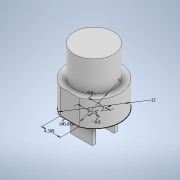
# Autodesk Inventor part: D6R90 F1 LFS
Saved by Autodesk Inventor 2021 (Build 250183000, 183)
## iProperties
Created: 2021-03-22
Part Number: D6R90 F1 LFS
Material: Generic
Document SubType Name: Modeling
Designer: ben
Density: 1 g/cm^3
Appearance: Default
Author: ben
Autodesk Inventor part; units mm, degrees
ref_plane "YZ Plane" through (0, 0, 0) normal (1, 0, 0) x (0, 1, 0)
ref_plane "XZ Plane" through (0, 0, 0) normal (0, 1, 0) x (-1, 0, 0)
ref_plane "XY Plane" through (0, 0, 0) normal (0, 0, 1) x (1, 0, 0)
sketch "Sketch1" plane through (0, 0, 0) normal (0, 1, 0) x (-1, 0, 0)
  arc A0 (-2.1541, 5.6) -> (2.1541, 5.6) centre (0, 0) ccw
  circle A1 centre (0, 0) radius 4.5
  line L0 (0, 5.6) -> (2.1541, 5.6)
  line L1 (0, 5.6) -> (-2.1541, 5.6)
  line L2 (0, 5.6) -> (3.5069, 5.6) construction
  line L3 (2.5, 2.9) -> (-2.5, 2.9)
  line L4 (-2.5, 2.9) -> (-2.5, 2.1)
  line L5 (-2.5, 2.1) -> (2.5, 2.1)
  line L6 (2.5, 2.1) -> (2.5, 2.9)
  line L7 (-2.5, -2.9) -> (2.5, -2.9)
  line L8 (2.5, -2.9) -> (2.5, -2.1)
  line L9 (2.5, -2.1) -> (-2.5, -2.1)
  line L10 (-2.5, -2.1) -> (-2.5, -2.9)
  line L11 (-2.5, 2.5) -> (2.5, 2.5)
  line L12 (-2.5, -2.5) -> (2.5, -2.5)
  line L13 (-4.5, 0) -> (4.5, 0)
  dimension "d0" = 12
  dimension "d1" = 9
  dimension "d2" = 180
  dimension "d3" = 4.3081
  dimension "d8" = 5
  dimension "d9" = 0.8
  dimension "d10" = 5
  dimension "d11" = 0.8
  dimension "d16" = 2.5
  dimension "d17" = 2.5
  constraints: 28 end point, 5 horizontal, 4 midpoint, 4 parallel, 4 point on circle, 2 centre point, 2 coincident, 2 perpendicular, 2 point on line
  measures "d0" diameter of A0
  measures "d1" diameter of A1
  measures "d2" angle of L1 L2
  measures "d3" distance of L0.end L1.end
  measures "d8" distance of L5.end L4.end
  measures "d9" distance of L4.end L3.end
  measures "d10" distance of L9.end L8.end
  measures "d11" distance of L8.end L7.end
  measures "d16" distance between parallel lines of L11 L13
  measures "d17" distance between parallel lines of L12 L13
extrude "Extrusion1" add sketch "Sketch1" along normal blind 5.8 contours L1 L0 A0
extrude "Extrusion2" add sketch "Sketch1" along normal blind 12.8 contours L13 A1 | A1 L13 | L6 L11 L4 L3 | L6 L5 L4 L11 | L10 L12 L8 L7 | L10 L9 L8 L12
extrude "Extrusion3" add sketch "Sketch1" against normal blind 5 contours L6 L11 L4 L3 | L6 L5 L4 L11 | L10 L12 L8 L7 | L10 L9 L8 L12
body "Solid1"
